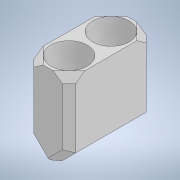
# Autodesk Inventor part: LineBig
Saved by Autodesk Inventor 2020 (Build 240168000, 168)
## iProperties
Created: 2020-02-13
Part Number: LineBig
Material: Generic
Document SubType Name: Modeling
Designer: atmat
Density: 1 g/cm^3
Appearance: Default
Author: atmat
Autodesk Inventor part; units mm, degrees
ref_plane "YZ Plane" through (0, 0, 0) normal (1, 0, 0) x (0, 1, 0)
ref_plane "XZ Plane" through (0, 0, 0) normal (0, 1, 0) x (-1, 0, 0)
ref_plane "XY Plane" through (0, 0, 0) normal (0, 0, 1) x (1, 0, 0)
sketch "Sketch1" plane through (0, 0, 0) normal (0, 1, 0) x (-1, 0, 0)
  circle A0 centre (0, 3.1667) radius 2.75
  circle A1 centre (0, -3.1333) radius 2.75
  line L0 (3.15, 6.3167) -> (-3.15, 6.3167)
  line L1 (-3.15, 6.3167) -> (-3.15, -6.2833)
  line L2 (-3.15, -6.2833) -> (3.15, -6.2833)
  line L3 (3.15, -6.2833) -> (3.15, 6.3167)
  point P0 (0, 0)
  dimension "d0" = 5.5
  dimension "d1" = 5.5
  dimension "d2" = 6.3
  dimension "d3" = 3.1667
  dimension "d4" = 3.15
  dimension "d5" = 3.15
  dimension "d6" = 3.15
  dimension "d7" = 3.15
  constraints: 8 end point, 2 centre point, 2 parallel, 1 horizontal, 1 perpendicular
  measures "d0" diameter of A0
  measures "d1" diameter of A1
  measures "d2" distance of A1.centre A0.centre
  measures "d3" distance of point (0, 0) A0.centre
  measures "d4" distance from line of L0 A0.centre
  measures "d5" distance from line of L2 A1.centre
  measures "d6" distance from line of L3 A1.centre
  measures "d7" distance from line of L1 A0.centre
extrude "Extrusion1" add sketch "Sketch1" along normal blind 10
sketch "Sketch2" plane through (3.15, 0, -6.2833) normal (0, 0, -1) x (-1, 0, 0)
  line L0 (0, 0) -> (0, 10) projected
  line L1 (0, 0) -> (6.3, 0)
  line L2 (6.3, 0) -> (0, 0) projected
  line L3 (0, 0) -> (3.15, -3.15)
  line L4 (3.15, -3.15) -> (6.3, 0)
  line L5 (6.3, 0) -> (0, 0)
  point P0 (3.15, 0)
  dimension "d11" = 45
  dimension "d12" = 45
  constraints: 8 end point, 1 horizontal, 1 perpendicular
  measures "d11" angle of L1 L4
  measures "d12" angle of L3 L1
extrude "Extrusion2" add sketch "Sketch2" against normal blind 12.6
sketch "Sketch3" plane through (0, 0, -3.1333) normal (0, 1, 0) x (1, 0, 0)
  line L0 (0, 3.15) -> (0, -9.45) projected
  circle A0 centre (0, 1.27) radius 1
  circle A1 centre (0, -1.27) radius 1
  circle A2 centre (0, -5.03) radius 1
  circle A3 centre (0, -7.57) radius 1
  circle A4 centre (0, -6.3) radius 2.75 projected
  circle A5 centre (0, 0) radius 2.75 projected
  point P0 (0, -3.1333)
  dimension "d15" = 2
  dimension "d16" = 2
  dimension "d17" = 2
  dimension "d18" = 2
  dimension "d19" = 2.54
  dimension "d20" = 2.54
  dimension "d21" = 1.27
  dimension "d22" = 1.27
  constraints: 4 centre point, 4 point on line
  measures "d15" diameter of A0
  measures "d16" diameter of A1
  measures "d17" diameter of A2
  measures "d18" diameter of A3
  measures "d19" distance of A0.centre A1.centre
  measures "d20" distance of A3.centre A2.centre
  measures "d21" distance of A4.centre A3.centre
  measures "d22" distance of A5.centre A1.centre
extrude "Extrusion3" cut sketch "Sketch3" against normal blind 4 contours A0 L0 | L0 A0 | A1 L0 | L0 A1 | A2 L0 | L0 A2 | A3 L0 | L0 A3
chamfer "Chamfer1" distance 1.5 angle 45 1 edges at (0, -3.15, -5.8433)
chamfer "Chamfer2" distance 1 angle 45 8 edges at (-3.15, 5, -6.2833) (3.15, 5, -6.2833) (3.15, 5, 6.3167) (-3.15, 5, 6.3167) (-2.1053, -1.0447, -6.2833) (2.1053, -1.0447, -6.2833) (2.1053, -1.0447, 6.3167) (-2.1053, -1.0447, 6.3167)
chamfer "Chamfer3" distance 1 angle 45 4 edges at (-2.65, 10, -5.7833) (2.65, 10, -5.7833) (2.65, 10, 5.8167) (-2.65, 10, 5.8167)
body "Solid1"
